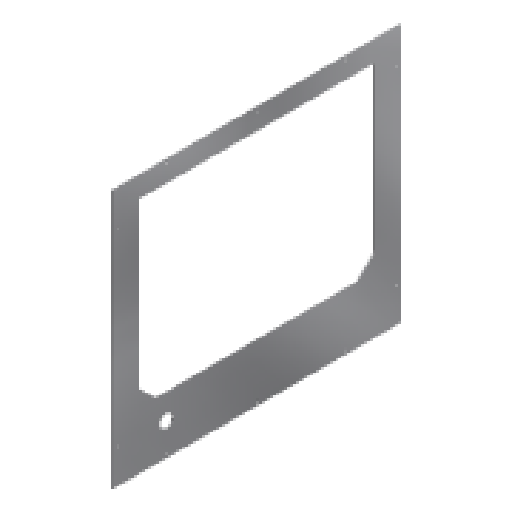
# Autodesk Inventor part: Front Panel
Saved by Autodesk Inventor 2023.2 (Build 272271000, 271)
## iProperties
Created: 2023-02-06
Part Number: Front Panel
Material: Aluminum 6061
Document SubType Name: Modeling
Designer: remop
Density: 2.7 g/cm^3
Appearance: Aluminum - Flat
Author: remop
Autodesk Inventor part; units mm, degrees
ref_plane "YZ Plane" through (0, 0, 0) normal (1, 0, 0) x (0, 1, 0)
ref_plane "XZ Plane" through (0, 0, 0) normal (0, 1, 0) x (-1, 0, 0)
ref_plane "XY Plane" through (0, 0, 0) normal (0, 0, 1) x (1, 0, 0)
sketch "Sketch1" plane through (0, 0, 0) normal (1, 0, 0) x (0, 1, 0)
  line L0 (465, 411) -> (465, -123) projected
  line L1 (465, -123) -> (-15, -123) projected
  line L2 (-15, -123) -> (-15, 411) projected
  line L3 (-15, 411) -> (465, 411) projected
  circle A0 centre (400, -113.5) radius 1.75 projected
  circle A1 centre (50, 401.5) radius 1.75 projected
  circle A2 centre (400, 401.5) radius 1.75 projected
  circle A3 centre (-7.5, -21) radius 1.75 projected
  circle A4 centre (-7.5, 144) radius 1.75 projected
  circle A5 centre (-7.5, 309) radius 1.75 projected
  circle A6 centre (457.5, 144) radius 1.75 projected
  circle A7 centre (457.5, -21) radius 1.75 projected
  circle A8 centre (457.5, 309) radius 1.75 projected
  circle A9 centre (50, -113.5) radius 1.75 projected
  point P0 (0, 0)
extrude "Extrusion1" add sketch "Sketch1" along normal blind 2
sketch "Sketch2" plane through (0, 0, 0) normal (-1, 0, 0) x (0, 0, 1)
  line L0 (411, -15) -> (-123, -15) projected
  line L1 (411, 465) -> (411, -15) projected
  line L2 (-123, 465) -> (411, 465) projected
  line L3 (-123, -15) -> (-123, 465) projected
  circle A0 centre (-113.5, 50) radius 1.75 projected
  circle A1 centre (-21, 457.5) radius 1.75 projected
  circle A2 centre (144, 457.5) radius 1.75 projected
  circle A3 centre (309, -7.5) radius 1.75 projected
  circle A4 centre (144, -7.5) radius 1.75 projected
  circle A5 centre (-21, -7.5) radius 1.75 projected
  circle A6 centre (401.5, 400) radius 1.75 projected
  circle A7 centre (401.5, 50) radius 1.75 projected
  circle A8 centre (-113.5, 400) radius 1.75 projected
  circle A9 centre (309, 457.5) radius 1.75 projected
  line L4 (-73, 425) -> (361, 425)
  line L5 (361, 425) -> (361, 92)
  line L6 (361, 92) -> (-73, 92)
  line L7 (-73, 92) -> (-73, 425)
  point P0 (0, 0)
  dimension "d2" = 50
  dimension "d3" = 50
  dimension "d4" = 40
  dimension "d5" = 107
  constraints: 8 end point, 2 parallel, 1 horizontal, 1 perpendicular
  measures "d2" distance between parallel lines of L3 L7
  measures "d3" distance between parallel lines of L1 L5
  measures "d4" distance between parallel lines of L2 L4
  measures "d5" distance between parallel lines of L0 L6
extrude "Extrusion2" cut sketch "Sketch2" against normal blind 2 contours L4 L5 L6 L7
chamfer "Chamfer1" distance 30 angle 45 2 edges at (1, 92, -73) (1, 92, 361)
sketch "Sketch3" plane through (0, 0, 0) normal (-1, 0, 0) x (0, 0, 1)
  line L0 (361, 425) -> (361, 122) projected
  line L1 (331, 92) -> (361, 122) projected
  line L2 (331, 92) -> (-43, 92) projected
  line L3 (-73, 122) -> (-43, 92) projected
  line L4 (-73, 122) -> (-73, 425) projected
  line L5 (-73, 425) -> (361, 425) projected
  line L6 (411, -15) -> (-123, -15) projected
  line L7 (411, 465) -> (411, -15) projected
  line L8 (-123, 465) -> (411, 465) projected
  line L9 (-123, -15) -> (-123, 465) projected
  circle A0 centre (-113.5, 50) radius 1.75 projected
  circle A1 centre (-21, 457.5) radius 1.75 projected
  circle A2 centre (144, 457.5) radius 1.75 projected
  circle A3 centre (309, -7.5) radius 1.75 projected
  circle A4 centre (144, -7.5) radius 1.75 projected
  circle A5 centre (-21, -7.5) radius 1.75 projected
  circle A6 centre (401.5, 400) radius 1.75 projected
  circle A7 centre (401.5, 50) radius 1.75 projected
  circle A8 centre (-113.5, 400) radius 1.75 projected
  circle A9 centre (309, 457.5) radius 1.75 projected
  circle A10 centre (311, 45) radius 11.5
  point P0 (0, 0)
  dimension "d11" = 23
  dimension "d12" = 60
  dimension "d13" = 100
  constraints: 1 centre point
  measures "d11" diameter of A10
  measures "d12" distance from line of L6 A10.centre
  measures "d13" distance from line of L7 A10.centre
extrude "Extrusion3" cut sketch "Sketch3" against normal through all contours A10
equation "\"d3\" = d2"
body "Solid1"
